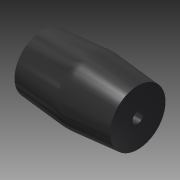
# Autodesk Inventor part: Rubber
Saved by Autodesk Inventor 2014 SP2 (Build 180246200, 246)
## iProperties
Created: 2019-06-15
Part Number: Rubber
Material: Generic
Document SubType Name: Modeling
Designer: Yuchofif
Density: 1 g/cm^3
Appearance: Default
Author: Yuchofif
Autodesk Inventor part; units mm, degrees
ref_plane "YZ Plane" through (0, 0, 0) normal (1, 0, 0) x (0, 1, 0)
ref_plane "XZ Plane" through (0, 0, 0) normal (0, 1, 0) x (-1, 0, 0)
ref_plane "XY Plane" through (0, 0, 0) normal (0, 0, 1) x (1, 0, 0)
sketch "Sketch1" plane through (0, 0, 0) normal (1, 0, 0) x (0, 1, 0)
  point P0 (0, 0)
sketch "Sketch2" plane through (0, 0, 0) normal (0, 0, 1) x (1, 0, 0)
  point P0 (0, 0)
sketch "Sketch3" plane through (0, 0, 0) normal (1, 0, 0) x (0, 1, 0)
  circle A0 centre (0, 0) radius 6
  constraints: 1 centre point, 1 coincident
extrude "Extrusion1" add sketch "Sketch3" along normal mid plane 18
sketch "Sketch4" plane through (0, 0, 0) normal (0, 0, 1) x (1, 0, 0)
  line L0 (-9, 6) -> (-9, -6) projected
  line L1 (9, -6) -> (9, 6) projected
  point P0 (0, 0)
sketch "Sketch5" plane through (9, 0, 0) normal (1, 0, 0) x (0, 0, -1)
  circle A0 centre (0, 0) radius 6 projected
  circle A1 centre (0, 0) radius 1
  constraints: 1 centre point, 1 coincident
extrude "Extrusion2" cut sketch "Sketch5" against normal blind 18 contours A1
chamfer "Chamfer1" distance 9 angle 5 1 edges at (9, -6, 0) measured on face at (8.5, -6, 0)
chamfer "Chamfer2" distance 9 angle 5 1 edges at (-9, -6, 0) measured on face at (-8.5, -6, 0)
fillet "Fillet1" radius 10 3 edges at (-0.0001, -6, 0) (0, -6, 0) (0.0001, -6, 0)
body "Solid1"
